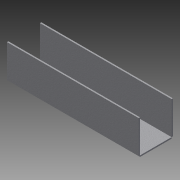
# Autodesk Inventor part: meera's skillz
Saved by Autodesk Inventor 2015 (Build 190159000, 159)
## iProperties
Created: 2014-11-14
Part Number: meera's skillz
Material: Generic
Document SubType Name: Modeling
Designer: srinis
Density: 1 g/cm^3
Appearance: Aluminum Cast
Author: srinis
Autodesk Inventor part; units mm, degrees
ref_plane "YZ Plane" through (0, 0, 0) normal (1, 0, 0) x (0, 1, 0)
ref_plane "XZ Plane" through (0, 0, 0) normal (0, 1, 0) x (-1, 0, 0)
ref_plane "XY Plane" through (0, 0, 0) normal (0, 0, 1) x (1, 0, 0)
sketch "Sketch1" plane through (0, 0, 0) normal (0, 1, 0) x (-1, 0, 0)
  line L0 (0, 0) -> (-304.8, 0)
  line L1 (-304.8, 0) -> (-304.8, -76.2)
  line L2 (-304.8, -76.2) -> (0, -76.2)
  line L3 (0, -76.2) -> (0, 0)
  line L4 (0, 0) -> (-304.8, 0)
  line L5 (-304.8, 0) -> (-304.8, -3.175)
  line L6 (-304.8, -3.175) -> (0, -3.175)
  line L7 (0, -3.175) -> (0, 0)
  line L8 (0, -76.2) -> (-304.8, -76.2)
  line L9 (-304.8, -76.2) -> (-304.8, -79.375)
  line L10 (-304.8, -79.375) -> (0, -79.375)
  line L11 (0, -79.375) -> (0, -76.2)
  dimension "d0" = 304.8
  dimension "d1" = 76.2
  dimension "d2" = 304.8
  dimension "d3" = 3.175
  dimension "d4" = 304.8
  dimension "d5" = 3.175
  constraints: 24 end point, 6 parallel, 3 horizontal, 3 perpendicular
  measures "d0" distance of L2.end L1.end
  measures "d1" distance of L1.end L0.end
  measures "d2" distance of L6.end L5.end
  measures "d3" distance of L5.end L4.end
  measures "d4" distance of L10.end L9.end
  measures "d5" distance of L9.end L8.end
extrude "Extrusion1" add sketch "Sketch1" along normal blind 3.175 contours L3 L2 L1 L6
sketch "Sketch2" plane through (0, 3.175, 0) normal (0, 1, 0) x (1, 0, 0)
  line L0 (0, 3.175) -> (304.8, 3.175)
  line L1 (304.8, 3.175) -> (304.8, 0)
  line L2 (304.8, 0) -> (0, 0)
  line L3 (0, 0) -> (0, 3.175)
  dimension "d8" = 304.8
  dimension "d9" = 3.175
  constraints: 8 end point, 2 parallel, 1 horizontal, 1 perpendicular
  measures "d8" distance of L1.end L2.end
  measures "d9" distance of L0.end L1.end
extrude "Extrusion2" add sketch "Sketch2" along normal blind 76.2
sketch "Sketch3" plane through (0, 3.175, 0) normal (0, 1, 0) x (1, 0, 0)
  line L0 (0, 76.2) -> (304.8, 76.2)
  line L1 (304.8, 76.2) -> (304.8, 79.375)
  line L2 (304.8, 79.375) -> (0, 79.375)
  line L3 (0, 79.375) -> (0, 76.2)
  point P0 (0, 0)
  dimension "d12" = 304.8
  dimension "d13" = 3.175
  constraints: 8 end point, 2 parallel, 1 horizontal, 1 perpendicular
  measures "d12" distance of L2.end L1.end
  measures "d13" distance of L1.end L0.end
extrude "Extrusion3" add sketch "Sketch3" along normal blind 76.2
body "Solid1"
